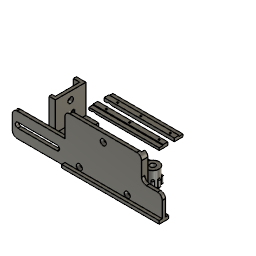
camera_steady (Autodesk Fusion 360 design; units mm, degrees)
Autodesk Fusion 360 part; units mm, degrees
sketch "Sketch1" plane through (0, 0, 0) normal (0, 0, 1) x (1, 0, 0)
  line L0 (-42, 80) -> (-26, 80)
  line L1 (0, 50) -> (118, 50)
  line L2 (118, 50) -> (118, 62)
  line L3 (118, 62) -> (-70, 62)
  line L4 (-70, 62) -> (-70, 54)
  line L5 (-4, 54) -> (-4, 62)
  line L6 (0, 54) -> (0, 62)
  line L7 (88, 50) -> (88, 62)
  line L8 (92, 50) -> (92, 62)
  line L9 (118, 58) -> (-70, 58)
  line L10 (-70, 54) -> (98, 54)
  line L11 (-42, 118.4) -> (-42, 80)
  line L12 (-26, 118.4) -> (-26, 80)
  line L13 (-42, 118.4) -> (-26, 118.4)
  line L14 (-42, 118.4) -> (-46, 118.4)
  line L15 (-42, 80) -> (-46, 80)
  line L16 (-46, 114.4) -> (-46, 84)
  line L17 (-46, 118.4) -> (-54, 118.4)
  line L18 (-46, 80) -> (-50, 80)
  line L19 (-46, 114.4) -> (-54, 114.4)
  line L20 (-46, 80) -> (-50, 80)
  line L21 (-46, 84) -> (-50, 84)
  line L22 (-54, 118.4) -> (-54, 114.4)
  line L23 (-50, 80) -> (-50, 84)
  line L24 (25, 80) -> (50, 80)
  line L25 (50, 80) -> (50, 110)
  line L26 (50, 110) -> (25, 110)
  line L27 (25, 84) -> (50, 84)
  circle A0 centre (35, 95) radius 3.2
  circle A1 centre (35, 95) radius 10.7
  line L28 (-50, 130) -> (36, 130)
  line L29 (36, 141) -> (-50, 141)
  line L30 (-50, 141) -> (-50, 130)
  line L31 (-50, 135) -> (36, 135)
  circle A2 centre (-36, 138) radius 1.1
  circle A3 centre (-7, 138) radius 1.1
  circle A4 centre (30, 138) radius 1.1
  line L32 (-50, 145) -> (35, 145) construction
  circle A5 centre (30, 152) radius 1.1
  line L33 (-50, 149) -> (-50, 160)
  line L34 (-50, 155) -> (36, 155)
  line L35 (36, 149) -> (-50, 149)
  circle A6 centre (-36, 152) radius 1.1
  line L36 (-50, 160) -> (36, 160)
  circle A7 centre (-7, 152) radius 1.1
  line L37 (-44, 141) -> (-44, 130)
  line L38 (-44, 149) -> (-44, 160)
  line L39 (98, 54) -> (118, 54)
  line L40 (20.0797, 95) -> (20.0797, 110)
  line L41 (20.0797, 95) -> (20.0797, 80)
  line L42 (25, 80) -> (20.0797, 80)
  line L43 (25, 84) -> (20.0797, 84)
  line L44 (25, 110) -> (20.0797, 110)
  line L45 (-4, 54) -> (-4, 50)
  line L46 (-4, 50) -> (0, 50)
  circle A8 centre (70, 90) radius 3.3
  circle A9 centre (70, 90) radius 8
  arc A10 (65.4986, 96.6134) -> (63.3866, 94.5014) centre (64.3431, 95.6569) ccw
  arc A11 (71.4934, 97.8594) -> (68.5066, 97.8594) centre (70, 98) ccw
  arc A12 (76.6134, 94.5014) -> (74.5014, 96.6134) centre (75.6569, 95.6569) ccw
  arc A13 (77.8594, 88.5066) -> (77.8594, 91.4934) centre (78, 90) ccw
  arc A14 (74.5014, 83.3866) -> (76.6134, 85.4986) centre (75.6569, 84.3431) ccw
  arc A15 (68.5066, 82.1406) -> (71.4934, 82.1406) centre (70, 82) ccw
  arc A16 (63.3866, 85.4986) -> (65.4986, 83.3866) centre (64.3431, 84.3431) ccw
  arc A17 (62.1406, 91.4934) -> (62.1406, 88.5066) centre (62, 90) ccw
  line L47 (38, 160) -> (38, 149)
  line L48 (36, 149) -> (38, 149)
  line L49 (36, 160) -> (38, 160)
  line L50 (36, 155) -> (38, 155)
  line L51 (38, 130) -> (38, 141)
  line L52 (36, 130) -> (38, 130)
  line L53 (36, 141) -> (38, 141)
  line L54 (36, 135) -> (38, 135)
  line L55 (35, 89.1571) -> (29.9399, 92.0785)
  line L56 (29.9399, 92.0785) -> (29.9399, 97.9215)
  line L57 (29.9399, 97.9215) -> (35, 100.8429)
  line L58 (35, 100.8429) -> (40.0601, 97.9215)
  line L59 (40.0601, 97.9215) -> (40.0601, 92.0785)
  line L60 (40.0601, 92.0785) -> (35, 89.1571)
  point P0 (35, 95)
  point P1 (-7, 141)
  point P2 (-7, 138)
  point P3 (-36, 138)
  point P4 (30, 138)
  point P5 (30, 152)
  point P6 (-7, 152)
  point P7 (-36, 152)
  point P8 (-7, 149)
  point P9 (-44, 130)
  point P10 (-44, 149)
  point P11 (70, 90)
  point P12 (70, 98)
  dimension "d43" = 168
  dimension "d54" = 38.4
  dimension "d64" = 4
  dimension "d69" = 4
  dimension "d81" = 6.4
  dimension "d82" = 21.4
  dimension "d92" = 86
  dimension "d93" = 11
  dimension "d100" = 2.2
  dimension "d101" = 2.2
  dimension "d102" = 2.2
  dimension "d103" = 11
  dimension "d118" = 6.6
  dimension "d119" = 16
  dimension "d120" = 3
  dimension "d122" = 360
  constraint horizontal L0
  constraint horizontal L1
  constraint vertical L2
  constraint horizontal L3
  constraint vertical L4
  constraint coincident L3 L5.end
  constraint perpendicular L3 L5
  constraint coincident L3 L6.end
  constraint perpendicular L3 L6
  constraint coincident L3 L7.end
  constraint perpendicular L3 L7
  constraint coincident L3 L8.end
  constraint perpendicular L3 L8
  constraint coincident L1 L7.start
  constraint coincident L1 L8.start
  constraint horizontal L9
  constraint horizontal L10
  constraint vertical L11
  constraint vertical L12
  constraint coincident L10 L5.start
  constraint perpendicular L12 L13
  constraint perpendicular L11 L14
  constraint perpendicular L11 L15
  constraint perpendicular L16 L17
  constraint perpendicular L16 L18
  constraint perpendicular L19 L22
  constraint perpendicular L21 L23
  constraint horizontal L24
  constraint vertical L25
  constraint horizontal L26
  constraint horizontal L27
  constraint coincident P0 A0.centre
  constraint concentric A0 A1
  constraint horizontal L28
  constraint horizontal L29
  constraint vertical L30
  constraint horizontal L31
  constraint midpoint L29 P1
  constraint coincident P3 A2.centre
  constraint coincident P2 A3.centre
  constraint coincident P4 A4.centre
  constraint horizontal L32
  constraint symmetric L28.start L32 L33.end
  constraint symmetric L28.end L32 L36.end
  constraint symmetric L29.start L32 L35.start
  constraint symmetric L29.end L32 L33.start
  constraint symmetric L31.start L32 L34.start
  constraint symmetric L31.end L32 L34.end
  constraint symmetric P1 L32 P8
  constraint symmetric P2 L32 P6
  constraint symmetric P3 L32 P7
  constraint symmetric P4 L32 P5
  constraint symmetric A2 L32 A6
  constraint symmetric A3 L32 A7
  constraint symmetric A4 L32 A5
  constraint vertical L37
  constraint coincident P9 L37.end
  constraint coincident P10 L38.start
  constraint coincident L2 L39.end
  constraint perpendicular L2 L39
  constraint midpoint L4 L9.end
  constraint perpendicular L41 L42
  constraint coincident L41 L43.end
  constraint perpendicular L41 L43
  constraint perpendicular L40 L44
  constraint perpendicular L10 L45
  constraint perpendicular L6 L46
  constraint coincident L10 L6.start
  constraint coincident P11 A8.centre
  constraint concentric A8 A9
  constraint coincident A9 P12
  constraint coincident P12 A11.centre
  constraint coincident A9 A10.end
  constraint coincident A9 A10.start
  constraint coincident A9 A11.end
  constraint coincident A9 A11.start
  constraint coincident A9 A12.end
  constraint coincident A9 A12.start
  constraint coincident A9 A13.end
  constraint coincident A9 A13.start
  constraint coincident A9 A14.end
  constraint coincident A9 A14.start
  constraint coincident A9 A15.end
  constraint coincident A9 A15.start
  constraint coincident A9 A16.end
  constraint coincident A9 A16.start
  constraint coincident A9 A17.end
  constraint coincident A9 A17.start
  constraint perpendicular L47 L48
  constraint perpendicular L47 L49
  constraint coincident L47 L50.end
  constraint perpendicular L47 L50
  constraint vertical L51
  constraint perpendicular L51 L52
  constraint perpendicular L51 L53
  constraint coincident L51 L54.end
  constraint perpendicular L51 L54
  measures "d43" distance of L10.end L4.end
  measures "d54" distance of L0.start L11.start
  measures "d64" distance of L0.start L15.end
  measures "d69" distance of L21.end L16.end
  measures "d81" diameter of A0
  measures "d82" diameter of A1
  measures "d92" distance of L28.start L28.end
  measures "d93" distance of L28.start L29.end
  measures "d100" diameter of A2
  measures "d101" diameter of A3
  measures "d102" diameter of A4
  measures "d103" distance of P9 L37.start
  measures "d118" diameter of A8
  measures "d119" diameter of A9
  measures "d120" diameter of A11
extrude "Extrude15" add sketch "Sketch1" along normal blind 4 contours L1 L7 L10 L45 L46 | L1 L7 L8 L10 | L1 L2 L8 L10 L39 | L6 L7 L9 L10 makes body 1
extrude "Extrude16" add sketch "Sketch1" along normal blind 30 contours L4 L5 L9 L10 | L2 L8 L9 L10 L39 bodies 1
extrude "Extrude31" add sketch "Sketch1" along normal blind 60 contours L6 L7 L9 L10 | L7 L8 L9 L10 | L5 L6 L9 L10 | L3 L7 L8 L9 | L3 L5 L6 L9 bodies 1
extrude "Extrude17" add sketch "Sketch1" along normal blind 4 contours L3 L6 L7 L9 | L3 L4 L5 L9 | L2 L3 L8 L9 bodies 1
sketch "Sketch2" plane through (0, 54, 0) normal (0, -1, 0) x (1, 0, 0)
  line L0 (118, 30) -> (92, 30)
  line L1 (-70, 30) -> (-70, 0)
  line L2 (-70, 0) -> (-4, 0)
  line L3 (-4, 4) -> (118, 4)
  line L4 (92, 30) -> (92, 60)
  line L5 (92, 60) -> (-4, 60)
  line L6 (-4, 60) -> (-4, 30)
  arc A0 (-63, 18.2) -> (-63, 11.8) centre (-63, 15) ccw
  line L7 (-11, 15) -> (-63, 15) construction
  line L8 (118, 4) -> (118, 30)
  line L9 (-4, 0) -> (-4, 4)
  line L10 (-4, 30) -> (-70, 30)
  line L11 (-63, 18.2) -> (-13.9988, 18.2)
  line L12 (-63, 11.8) -> (-14, 11.8)
  line L13 (-4, 4) -> (-4, 60)
  line L14 (-4, 4) -> (-4, 60)
  line L15 (-4, 4) -> (-4, 60)
  arc A1 (-14, 11.8) -> (-14.0012, 18.2) centre (-14, 15) ccw
  circle A2 centre (74, 8) radius 1.3
  circle A3 centre (44, 50) radius 1.3
  circle A4 centre (14, 8) radius 1.3
  point P0 (-70, 15)
  point P1 (-225, 15)
  point P2 (-285, 15)
  point P3 (-37, 15)
  point P4 (-37, 15)
  point P5 (-21, 15)
  point P6 (-63, 15)
  point P7 (-14, 15)
  point P8 (44, 50)
  point P9 (44, 50)
  point P10 (49.3141, -3.6655)
  point P11 (14, 8)
  point P12 (74, 8)
  dimension "d115" = 6.4
  dimension "d135" = 6.4
  dimension "d147" = 2.6
  dimension "d148" = 2.6
  dimension "d149" = 2.6
  constraint midpoint L1 P0
  constraint horizontal L7
  constraint coincident P4 P3
  constraint midpoint L7 P4
  constraint coincident P6 A0.centre
  constraint parallel L10 L11
  constraint parallel L7 L12
  constraint coincident L7 P7
  constraint coincident P7 A1.centre
  constraint coincident L11.end A1
  constraint coincident L11 A1.end
  constraint coincident P12 A2.centre
  constraint coincident P9 P8
  constraint coincident P11 A4.centre
  measures "d115" diameter of A0
  measures "d135" diameter of A1
  measures "d147" diameter of A2
  measures "d148" diameter of A3
  measures "d149" diameter of A4
extrude "Extrude18" cut sketch "Sketch2" against normal blind 4 contours A0 L11 L12 A1 | A2 | A3 | A4 bodies 1
chamfer "Chamfer1" distance 2.4 angle 45 3 edges at (42.788, 54, 50.4701) (12.788, 54, 8.4701) (72.788, 54, 8.4701) on bodies 1
fillet "Fillet1" radius 6 6 edges at (92, 58, 60) (-4, 58, 60) (118, 56, 30) (92, 56, 30) (-70, 56, 30) (-70, 58, 0) on bodies 1
extrude "Extrude22" add sketch "Sketch1" along normal blind 4 separate body contours L0 L11 L12 L13 makes body 2
extrude "Extrude23" add sketch "Sketch1" along normal blind 40 contours L11 L14 L15 L16 L17 L18 L19 L20 L21 L22 L23 bodies 2
sketch "Sketch4" plane through (-42, 0, 0) normal (1, 0, 0) x (0, 1, 0)
  line L0 (80, 4) -> (118.4, 4)
  line L1 (118.4, 4) -> (118.4, 40)
  line L2 (118.4, 40) -> (80, 40)
  line L3 (80, 40) -> (80, 4)
  circle A0 centre (99.2, 30) radius 3.4
  circle A1 centre (99.2, 14) radius 3.4
  point P0 (99.2, 30)
  point P1 (99.2, 14)
  dimension "d87" = 6.8
  dimension "d88" = 6.8
  constraint coincident P0 A0.centre
  constraint coincident P1 A1.centre
  measures "d87" diameter of A0
  measures "d88" diameter of A1
extrude "Extrude24" cut sketch "Sketch4" against normal blind 4 contours A0 | A1 bodies 2
extrude "Extrude25" add sketch "Sketch1" along normal blind 4 separate body contours L25 L26 L27 L40 L41 L43 L44 makes body 3
extrude "Extrude26" add sketch "Sketch1" along normal blind 9 contours A1 | L55 L56 L57 L58 L59 L60 bodies 3
extrude "Extrude27" add sketch "Sketch1" along normal blind 9 contours A1 | L55 L56 L57 L58 L59 L60 bodies 3
sketch "Sketch7" plane through (0, 0, 9) normal (0, 0, 1) x (-1, 0, 0)
  circle A0 centre (-35, -95) radius 10.7
  circle A1 centre (-35, -95) radius 3.2
  line L0 (-40.0601, -92.0785) -> (-35, -89.1571)
  line L1 (-35, -89.1571) -> (-29.9399, -92.0785)
  line L2 (-29.9399, -92.0785) -> (-29.9399, -97.9215)
  line L3 (-29.9399, -97.9215) -> (-35, -100.8429)
  line L4 (-35, -100.8429) -> (-40.0601, -97.9215)
  line L5 (-40.0601, -97.9215) -> (-40.0601, -92.0785)
extrude "Extrude36" cut sketch "Sketch7" against normal blind 5 contours L0 L1 L2 L3 L4 L5 bodies 3
extrude "Extrude28" add sketch "Sketch1" along normal blind 4 separate body contours L29 L30 L31 L37 | L29 L31 L37 L51 L53 L54 | L33 L34 L35 L38 | L34 L35 L38 L47 L48 L50 makes body 4 at (-45.7, 138, 0) makes body 5 at (-45.7, 152, 0)
extrude "Extrude29" add sketch "Sketch1" along normal blind 3 contours L28 L30 L31 L37 | L28 L31 L37 L51 L52 L54 | L33 L34 L36 L38 | L34 L36 L38 L47 L49 L50 bodies 4 5
sketch "Sketch5" plane through (0, 130, 0) normal (0, -1, 0) x (1, 0, 0)
  line L0 (-50, 0) -> (38, 0)
  line L1 (38, 3) -> (-50, 3)
  line L2 (-50, 3) -> (-50, 0)
  arc A0 (-41.7579, 0) -> (-46.23, 0) centre (-43.9939, -2) ccw
  line L3 (38, 0) -> (38, 3)
  point P0 (-41.7579, 0)
  dimension "d107" = 6
  constraint coincident L0 A0.end
  constraint coincident L0 P0
  constraint coincident P0 A0.start
  measures "d107" diameter of A0
extrude "Extrude30" cut sketch "Sketch5" against normal blind 30 contours L0 A0 bodies 4 5
fillet "Fillet2" radius 2 4 edges at (50, 110, 2) (50, 84, 2) (20.0797, 110, 2) (20.0797, 84, 2) on bodies 3
extrude "Extrude32" add sketch "Sketch1" along normal blind 20 separate body contours A9 makes body 6
extrude "Extrude33" add sketch "Sketch1" along normal blind 10 contours A9 A13 | A9 A12 | A9 A14 | A9 A11 | A9 A15 | A9 A10 | A9 A16 | A9 A17 bodies 6
fillet "Fillet3" radius 1 8 edges at (76.7175, 96.7175, 10) (70, 99.5, 10) (63.2825, 96.7175, 10) (60.5, 90, 10) (63.2825, 83.2825, 10) (70, 80.5, 10) (76.7175, 83.2825, 10) (79.5, 90, 10) on bodies 6
fillet "Fillet4" radius 1 16 edges at (79.5, 90, 0) (76.7175, 96.7175, 0) (70, 99.5, 0) (63.2825, 96.7175, 0) (60.5, 90, 0) (63.2825, 83.2825, 0) (70, 80.5, 0) (76.7175, 83.2825, 0) (77.391, 93.0615, 0) (73.0615, 97.391, 0) (66.9385, 97.391, 0) (62.609, 93.0615, 0) (62.609, 86.9385, 0) (66.9385, 82.609, 0) (73.0615, 82.609, 0) (77.391, 86.9385, 0) on bodies 6
sketch "Sketch6" plane through (0, 0, 0) normal (0, 0, 1) x (1, 0, 0)
  line L0 (75.0701, 92.9272) -> (70, 95.8545)
  line L1 (70, 95.8545) -> (64.9299, 92.9272)
  line L2 (64.9299, 92.9272) -> (64.9299, 87.0728)
  line L3 (64.9299, 87.0728) -> (70, 84.1455)
  line L4 (70, 84.1455) -> (75.0701, 87.0728)
  line L5 (75.0701, 92.9272) -> (75.0701, 87.0728)
  point P0 (70, 90)
extrude "Extrude34" cut sketch "Sketch6" along normal blind 4 bodies 6
